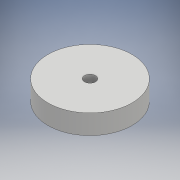
# Autodesk Inventor part: slipring
Saved by Autodesk Inventor 2017 (Build 210142000, 142)
## iProperties
Created: 2017-04-28
Part Number: slipring
Material: Generic
Document SubType Name: Modeling
Designer: s4321966
Density: 1 g/cm^3
Appearance: Default
Author: s4321966
Autodesk Inventor part; units mm, degrees
ref_plane "YZ Plane" through (0, 0, 0) normal (1, 0, 0) x (0, 1, 0)
ref_plane "XZ Plane" through (0, 0, 0) normal (0, 1, 0) x (-1, 0, 0)
ref_plane "XY Plane" through (0, 0, 0) normal (0, 0, 1) x (1, 0, 0)
sketch "Sketch1" plane through (0, 0, 0) normal (1, 0, 0) x (0, 1, 0)
  line L0 (0, 0) -> (18.9969, 0)
  line L1 (18.9969, 0) -> (18.9969, -8.8659)
  line L2 (18.9969, -8.8659) -> (0, -8.8659)
  line L3 (0, -8.8659) -> (0, 0)
  line L4 (0, 0) -> (2.5, 0)
  line L5 (2.5, 0) -> (2.5, -8.8659)
  dimension "d0" = 2.5
  constraints: 12 end point, 2 parallel, 2 perpendicular, 2 point on line, 1 horizontal
  measures "d0" distance of L0.start L4.end
revolve "Revolution1" add sketch "Sketch1" angle 360 about axis through (0, 0, -8.8659) along (0, 0, 1) contours L0 L1 L2 L5
body "Solid1"
